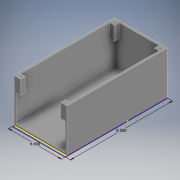
# Autodesk Inventor part: Part1
Saved by Autodesk Inventor 2021 (Build 250183000, 183)
## iProperties
Created: 2023-01-12
Part Number: Part1
Material: Generic
Document SubType Name: Modeling
Designer: boyle
Density: 1 g/cm^3
Appearance: Default
Author: boyle
Autodesk Inventor part; units mm, degrees
ref_plane "YZ Plane" through (0, 0, 0) normal (1, 0, 0) x (0, 1, 0)
ref_plane "XZ Plane" through (0, 0, 0) normal (0, 1, 0) x (-1, 0, 0)
ref_plane "XY Plane" through (0, 0, 0) normal (0, 0, 1) x (1, 0, 0)
sketch "Sketch1" plane through (0, 0, 0) normal (0, 1, 0) x (-1, 0, 0)
  line L0 (0, 0) -> (-111.76, 0)
  line L1 (-111.76, 0) -> (-111.76, 215.9)
  line L2 (-111.76, 215.9) -> (0, 215.9)
  line L3 (0, 215.9) -> (0, 0)
  dimension "d0" = 111.76
  dimension "d1" = 215.9
  constraints: 8 end point, 2 parallel, 1 horizontal, 1 perpendicular
  measures "d0" distance of L1.end L2.end
  measures "d1" distance of L0.end L1.end
extrude "Extrusion1" add sketch "Sketch1" along normal blind 91.44
shell "Shell1" thickness 3.81 removed faces 1 at (37.2533, 91.44, 71.9667)
sketch "Sketch2" plane through (0, 0, 215.9) normal (0, 0, 1) x (1, 0, 0)
  line L0 (0, 0) -> (111.76, 0) projected
  line L1 (111.76, 0) -> (111.76, 91.44) projected
  line L2 (0, 91.44) -> (111.76, 91.44) projected
  line L3 (0, 0) -> (0, 91.44) projected
  point P0 (0, 0)
extrude "Extrusion2" cut sketch "Sketch2" against normal up to surface (3.81 mm away)
sketch "Sketch3" plane through (0, 0, 0) normal (0, -1, 0) x (1, 0, 0)
  line L0 (111.76, 212.09) -> (0, 212.09) projected
  line L1 (0, 0) -> (0, 212.09) projected
  line L2 (111.76, 212.09) -> (111.76, 0) projected
  line L3 (111.76, 212.09) -> (0, 212.09) projected
  line L4 (0, 0) -> (0, 212.09) projected
  line L5 (111.76, 0) -> (0, 0) projected
  line L6 (111.76, 212.09) -> (111.76, 0) projected
  line L7 (111.76, 212.09) -> (111.76, 0) projected
  line L8 (0, 0) -> (0, 212.09) projected
  spline S0 degree 4 poles (111.76, 85.3366) (95.0927, 139.8259) (66.5153, -13.509) (18.6749, 203.0999) (15.6726, 63.615) (0, 106.045) knots 0 0 0 0 0 0.532853 1 1 1 1 1
  point P0 (85.9461, 95.2827)
  point P1 (57.1117, 86.6573)
  point P2 (28.3059, 111.5489)
  point P3 (15.0905, 97.7863)
  point P4 (0, 106.045)
  point P5 (111.76, 85.3366)
  constraints: 1 midpoint, 1 point on line, 6 other
sketch "Sketch4" plane through (0, 91.44, 0) normal (0, 1, 0) x (1, 0, 0)
  line L0 (3.81, -212.09) -> (3.81, -3.81) projected
  line L1 (3.81, -3.81) -> (107.95, -3.81) projected
  line L2 (107.95, -3.81) -> (107.95, -212.09) projected
  line L3 (107.95, -3.81) -> (3.81, -3.81) projected
  line L4 (3.81, -3.81) -> (13.81, -3.81)
  line L5 (13.81, -3.81) -> (13.81, -13.81)
  line L6 (13.81, -13.81) -> (3.81, -13.81)
  line L7 (3.81, -13.81) -> (3.81, -3.81)
  line L8 (107.95, -3.81) -> (97.95, -3.81)
  line L9 (97.95, -3.81) -> (97.95, -13.81)
  line L10 (97.95, -13.81) -> (107.95, -13.81)
  line L11 (107.95, -13.81) -> (107.95, -3.81)
  line L12 (107.95, -212.09) -> (107.95, -3.81) projected
  line L13 (107.95, -212.09) -> (97.95, -212.09)
  line L14 (97.95, -212.09) -> (97.95, -202.09)
  line L15 (97.95, -202.09) -> (107.95, -202.09)
  line L16 (107.95, -202.09) -> (107.95, -212.09)
  line L17 (3.81, -212.09) -> (13.81, -212.09)
  line L18 (13.81, -212.09) -> (13.81, -202.09)
  line L19 (13.81, -202.09) -> (3.81, -202.09)
  line L20 (3.81, -202.09) -> (3.81, -212.09)
  point P0 (3.81, -202.09)
  point P1 (97.95, -3.81)
  dimension "d9" = 10
  dimension "d10" = 10
  dimension "d11" = 10
  dimension "d12" = 10
  dimension "d13" = 10
  dimension "d14" = 10
  dimension "d15" = 10
  dimension "d16" = 10
  constraints: 32 end point, 8 parallel, 4 horizontal, 4 perpendicular
  measures "d9" distance of L5.end L6.end
  measures "d10" distance of L4.end L5.end
  measures "d11" distance of L10.end L9.end
  measures "d12" distance of L9.end L8.end
  measures "d13" distance of L14.end L15.end
  measures "d14" distance of L13.end L14.end
  measures "d15" distance of L19.end L18.end
  measures "d16" distance of L18.end L17.end
extrude "Extrusion4" add sketch "Sketch4" against normal blind 30
sketch "Sketch5" plane through (0, 91.44, 0) normal (0, 1, 0) x (1, 0, 0)
  circle A0 centre (8.81, -8.81) radius 2
  circle A1 centre (105.49, -8.81) radius 2
  circle A2 centre (105.49, -207.09) radius 2
  circle A3 centre (8.81, -207.09) radius 2
  dimension "d19" = 4
  dimension "d20" = 4
  dimension "d21" = 4
  dimension "d22" = 4
  constraints: 4 centre point
  measures "d19" diameter of A0
  measures "d20" diameter of A1
  measures "d21" diameter of A2
  measures "d22" diameter of A3
extrude "Extrusion5" cut sketch "Sketch5" against normal blind 15
body "Solid1"
